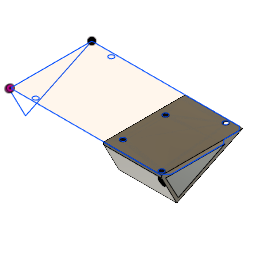
arduno wedge v1 (Autodesk Fusion 360 design; units mm, degrees)
Autodesk Fusion 360 part; units mm, degrees
(part 1 of 2)
sketch "dimensioniMega" plane through (-257.4607, -81.6493, 0) normal (0, 0, 1) x (1, 0, 0)
  line L0 (356.4838, 123.144) -> (359.0229, 120.6049)
  line L1 (359.0229, 120.6049) -> (359.0229, 86.3482)
  line L2 (258.4956, 82.5395) -> (258.2417, 82.5818)
  line L3 (258.2417, 82.5818) -> (258.0089, 82.6665)
  line L4 (258.4956, 135.8395) -> (353.9447, 135.8395)
  line L5 (257.7973, 135.5433) -> (258.0089, 135.6914)
  line L6 (356.4838, 133.3004) -> (356.4838, 123.144)
  line L7 (355.9971, 82.6665) -> (355.7432, 82.5818)
  line L8 (257.7973, 82.8357) -> (257.6281, 83.0473)
  line L9 (257.5434, 83.2801) -> (257.5011, 83.534)
  line L10 (359.0229, 86.3482) -> (356.4838, 83.8091)
  line L11 (355.4893, 82.5395) -> (258.4956, 82.5395)
  line L12 (257.5434, 135.0989) -> (257.6281, 135.3317)
  line L13 (258.0089, 135.6914) -> (258.2417, 135.7972)
  line L14 (257.5011, 134.8239) -> (257.5434, 135.0989)
  line L15 (257.6281, 135.3317) -> (257.7973, 135.5433)
  line L16 (356.4626, 83.2801) -> (356.3568, 83.0473)
  line L17 (356.4838, 83.8091) -> (356.4838, 83.534)
  line L18 (355.7432, 82.5818) -> (355.4893, 82.5395)
  line L19 (356.4838, 83.534) -> (356.4626, 83.2801)
  line L20 (258.0089, 82.6665) -> (257.7973, 82.8357)
  line L21 (258.2417, 135.7972) -> (258.4956, 135.8395)
  line L22 (257.5011, 83.534) -> (257.5011, 134.8239)
  line L23 (356.3568, 83.0473) -> (356.2087, 82.8357)
  line L24 (353.9447, 135.8395) -> (356.4838, 133.3004)
  line L25 (257.6281, 83.0473) -> (257.5434, 83.2801)
  line L26 (356.2087, 82.8357) -> (355.9971, 82.6665)
  line L27 (269.889, 85.3923) -> (269.879, 85.3375)
  line L28 (272.1711, 83.6333) -> (272.2211, 83.6587)
  line L29 (271.9631, 83.5492) -> (272.0162, 83.5675)
  line L30 (271.5223, 83.4715) -> (271.5783, 83.4744)
  line L31 (274.3429, 133.3561) -> (274.34, 133.4118)
  line L32 (271.3548, 83.4744) -> (271.4105, 83.4715)
  line L33 (274.3197, 133.5776) -> (274.3092, 133.6323)
  line L34 (273.0586, 84.8548) -> (273.0655, 84.9105)
  line L35 (274.3092, 133.6323) -> (274.2967, 133.6866)
  line L36 (274.2284, 133.8986) -> (274.2068, 133.95)
  line L37 (274.3284, 133.5226) -> (274.3197, 133.5776)
  line L38 (271.1342, 83.5051) -> (271.189, 83.4946)
  line L39 (272.7993, 84.1794) -> (272.8299, 84.2265)
  line L40 (272.1202, 83.6095) -> (272.1711, 83.6333)
  line L41 (270.1718, 84.1244) -> (270.2056, 84.0801)
  line L42 (269.9667, 85.6595) -> (269.9474, 85.6072)
  line L43 (273.0655, 84.9105) -> (273.0703, 84.9664)
  line L44 (271.189, 83.4946) -> (271.244, 83.4859)
  line L45 (272.2702, 83.686) -> (272.3183, 83.7149)
  line L46 (272.9115, 84.3737) -> (272.9352, 84.4245)
  line L47 (272.9956, 84.5817) -> (273.012, 84.6354)
  line L48 (274.34, 133.4118) -> (274.3351, 133.4673)
  line L49 (273.012, 84.6354) -> (273.0265, 84.6896)
  line L50 (272.8299, 84.2265) -> (272.8588, 84.2746)
  line L51 (273.0703, 84.9664) -> (273.0733, 85.0225)
  line L52 (273.0498, 84.7994) -> (273.0586, 84.8548)
  line L53 (272.5832, 83.9218) -> (272.6229, 83.9615)
  line L54 (272.6612, 84.0026) -> (272.698, 84.045)
  line L55 (273.0733, 85.0225) -> (273.0743, 85.0786)
  line L56 (271.7454, 83.4949) -> (271.8005, 83.5057)
  line L57 (271.244, 83.4859) -> (271.2993, 83.4792)
  line L58 (274.2824, 133.7405) -> (274.2663, 133.7938)
  line L59 (271.4105, 83.4715) -> (271.4662, 83.4705)
  line L60 (274.2663, 133.7938) -> (274.2482, 133.8465)
  line L61 (272.9773, 84.5286) -> (272.9956, 84.5817)
  line L62 (271.69, 83.4862) -> (271.7454, 83.4949)
  line L63 (272.5422, 83.8836) -> (272.5832, 83.9218)
  line L64 (271.6343, 83.4793) -> (271.69, 83.4862)
  line L65 (272.886, 84.3237) -> (272.9115, 84.3737)
  line L66 (271.0799, 83.5176) -> (271.1342, 83.5051)
  line L67 (272.4998, 83.8467) -> (272.5422, 83.8836)
  line L68 (273.0265, 84.6896) -> (273.0391, 84.7443)
  line L69 (272.2211, 83.6587) -> (272.2702, 83.686)
  line L70 (272.9572, 84.4762) -> (272.9773, 84.5286)
  line L71 (272.7671, 84.1334) -> (272.7993, 84.1794)
  line L72 (271.5783, 83.4744) -> (271.6343, 83.4793)
  line L73 (270.6196, 83.7114) -> (270.6675, 83.6829)
  line L74 (274.2967, 133.6866) -> (274.2824, 133.7405)
  line L75 (272.4562, 83.8114) -> (272.4998, 83.8467)
  line L76 (269.8688, 84.8933) -> (269.8762, 84.8381)
  line L77 (270.9728, 83.5481) -> (271.0261, 83.5319)
  line L78 (272.8588, 84.2746) -> (272.886, 84.3237)
  line L79 (272.7334, 84.0886) -> (272.7671, 84.1334)
  line L80 (274.3438, 133.3004) -> (274.3429, 133.3561)
  line L81 (274.3351, 133.4673) -> (274.3284, 133.5226)
  line L82 (271.2993, 83.4792) -> (271.3548, 83.4744)
  line L83 (272.698, 84.045) -> (272.7334, 84.0886)
  line L84 (272.4114, 83.7776) -> (272.4562, 83.8114)
  line L85 (273.0391, 84.7443) -> (273.0498, 84.7994)
  line L86 (272.3654, 83.7454) -> (272.4114, 83.7776)
  line L87 (271.8552, 83.5183) -> (271.9094, 83.5328)
  line L88 (271.9094, 83.5328) -> (271.9631, 83.5492)
  line L89 (271.0261, 83.5319) -> (271.0799, 83.5176)
  line L90 (273.6899, 134.5948) -> (273.6445, 134.6271)
  line L91 (273.6445, 134.6271) -> (273.598, 134.6578)
  line L92 (271.7227, 134.5494) -> (271.6801, 134.5135)
  line L93 (273.8191, 134.4888) -> (273.7773, 134.5256)
  line L94 (272.3183, 83.7149) -> (272.3654, 83.7454)
  line L95 (271.4662, 83.4705) -> (271.5223, 83.4715)
  line L96 (271.3884, 134.1783) -> (271.3588, 134.1311)
  line L97 (272.6229, 83.9615) -> (272.6612, 84.0026)
  line L98 (271.5599, 134.3974) -> (271.5226, 134.356)
  line L99 (274.1315, 134.0991) -> (274.103, 134.147)
  line L100 (272.4768, 134.8875) -> (272.422, 134.8776)
  line L101 (273.14, 134.8569) -> (273.0858, 134.8699)
  line L102 (272.532, 134.8955) -> (272.4768, 134.8875)
  line L103 (273.5505, 134.6868) -> (273.5019, 134.7142)
  line L104 (272.81, 134.9068) -> (272.7543, 134.9084)
  line L105 (274.2482, 133.8465) -> (274.2284, 133.8986)
  line L106 (272.0686, 83.5876) -> (272.1202, 83.6095)
  line L107 (271.3588, 134.1311) -> (271.3308, 134.0829)
  line L108 (273.8988, 134.4109) -> (273.8596, 134.4506)
  line L109 (272.9352, 84.4245) -> (272.9572, 84.4762)
  line L110 (271.3308, 134.0829) -> (271.3046, 134.0338)
  line L111 (271.3046, 134.0338) -> (271.28, 133.9838)
  line L112 (273.9729, 134.3277) -> (273.9366, 134.37)
  line L113 (271.6387, 134.4762) -> (271.5986, 134.4375)
  line L114 (273.8596, 134.4506) -> (273.8191, 134.4888)
  line L115 (272.5873, 134.9016) -> (272.532, 134.8955)
  line L116 (272.26, 134.8365) -> (272.2071, 134.8191)
  line L117 (272.0162, 83.5675) -> (272.0686, 83.5876)
  line L118 (273.5019, 134.7142) -> (273.4525, 134.7399)
  line L119 (271.905, 134.6773) -> (271.8578, 134.6477)
  line L120 (273.4525, 134.7399) -> (273.4022, 134.7639)
  line L121 (274.0411, 134.2396) -> (274.0077, 134.2843)
  line L122 (273.7342, 134.561) -> (273.6899, 134.5948)
  line L123 (272.0023, 134.7315) -> (271.9532, 134.7053)
  line L124 (273.2468, 134.8251) -> (273.1936, 134.8419)
  line L125 (272.3675, 134.8658) -> (272.3135, 134.8521)
  line L126 (271.5226, 134.356) -> (271.4868, 134.3134)
  line L127 (273.9366, 134.37) -> (273.8988, 134.4109)
  line L128 (272.6429, 134.9058) -> (272.5873, 134.9016)
  line L129 (271.7666, 134.5837) -> (271.7227, 134.5494)
  line L130 (272.1032, 134.7789) -> (272.0524, 134.7561)
  line L131 (271.8117, 134.6165) -> (271.7666, 134.5837)
  line L132 (273.7773, 134.5256) -> (273.7342, 134.561)
  line L133 (272.9763, 134.8904) -> (272.921, 134.8978)
  line L134 (272.8656, 134.9033) -> (272.81, 134.9068)
  line L135 (272.6986, 134.9081) -> (272.6429, 134.9058)
  line L136 (274.0077, 134.2843) -> (273.9729, 134.3277)
  line L137 (271.8005, 83.5057) -> (271.8552, 83.5183)
  line L138 (273.2993, 134.8065) -> (273.2468, 134.8251)
  line L139 (274.2068, 133.95) -> (274.1834, 134.0005)
  line L140 (272.0524, 134.7561) -> (272.0023, 134.7315)
  line L141 (273.4022, 134.7639) -> (273.3511, 134.7861)
  line L142 (272.3135, 134.8521) -> (272.26, 134.8365)
  line L143 (274.0728, 134.1938) -> (274.0411, 134.2396)
  line L144 (274.1834, 134.0005) -> (274.1583, 134.0503)
  line L145 (272.921, 134.8978) -> (272.8656, 134.9033)
  line L146 (274.1583, 134.0503) -> (274.1315, 134.0991)
  line L147 (272.2071, 134.8191) -> (272.1548, 134.7999)
  line L148 (271.9532, 134.7053) -> (271.905, 134.6773)
  line L149 (272.7543, 134.9084) -> (272.6986, 134.9081)
  line L150 (272.1548, 134.7999) -> (272.1032, 134.7789)
  line L151 (274.103, 134.147) -> (274.0728, 134.1938)
  line L152 (273.1936, 134.8419) -> (273.14, 134.8569)
  line L153 (271.8578, 134.6477) -> (271.8117, 134.6165)
  line L154 (271.5986, 134.4375) -> (271.5599, 134.3974)
  line L155 (273.0858, 134.8699) -> (273.0312, 134.8811)
  line L156 (271.4868, 134.3134) -> (271.4524, 134.2695)
  line L157 (272.422, 134.8776) -> (272.3675, 134.8658)
  line L158 (271.4524, 134.2695) -> (271.4196, 134.2245)
  line L159 (271.4196, 134.2245) -> (271.3884, 134.1783)
  line L160 (273.0312, 134.8811) -> (272.9763, 134.8904)
  line L161 (273.3511, 134.7861) -> (273.2993, 134.8065)
  line L162 (273.598, 134.6578) -> (273.5505, 134.6868)
  line L163 (271.6801, 134.5135) -> (271.6387, 134.4762)
  line L164 (271.5105, 132.2589) -> (271.5473, 132.217)
  line L165 (271.7084, 132.0632) -> (271.7519, 132.0284)
  line L166 (273.1248, 131.7401) -> (273.179, 131.7546)
  line L167 (271.1345, 133.4488) -> (271.1303, 133.3932)
  line L168 (272.9038, 131.7011) -> (272.9595, 131.708)
  line L169 (272.5136, 131.7077) -> (272.5689, 131.701)
  line L170 (272.5689, 131.701) -> (272.6244, 131.6962)
  line L171 (271.211, 132.7894) -> (271.2296, 132.7369)
  line L172 (271.7519, 132.0284) -> (271.7965, 131.9951)
  line L173 (271.8892, 131.9332) -> (271.937, 131.9047)
  line L174 (271.184, 133.7226) -> (271.1703, 133.6686)
  line L175 (271.5856, 132.1765) -> (271.6252, 132.1374)
  line L176 (271.1662, 132.9503) -> (271.1793, 132.8962)
  line L177 (271.1293, 133.2261) -> (271.1329, 133.1705)
  line L178 (271.3784, 132.4381) -> (271.409, 132.3916)
  line L179 (271.8423, 131.9633) -> (271.8892, 131.9332)
  line L180 (272.2956, 131.7537) -> (272.3495, 131.7394)
  line L181 (272.8479, 131.6962) -> (272.9038, 131.7011)
  line L182 (271.1793, 132.8962) -> (271.1942, 132.8425)
  line L183 (271.6252, 132.1374) -> (271.6661, 132.0996)
  line L184 (271.1303, 133.3932) -> (271.128, 133.3376)
  line L185 (271.1383, 133.1151) -> (271.1457, 133.0599)
  line L186 (271.1486, 133.5593) -> (271.1406, 133.5042)
  line L187 (271.128, 133.3376) -> (271.1277, 133.2818)
  line L188 (272.4038, 131.7269) -> (272.4585, 131.7164)
  line L189 (272.0862, 131.8293) -> (272.1375, 131.8077)
  line L190 (271.28, 133.9838) -> (271.2572, 133.9329)
  line L191 (271.1277, 133.2818) -> (271.1293, 133.2261)
  line L192 (271.2722, 132.6339) -> (271.2962, 132.5836)
  line L193 (271.5473, 132.217) -> (271.5856, 132.1765)
  line L194 (271.9859, 131.8778) -> (272.0356, 131.8527)
  line L195 (271.6661, 132.0996) -> (271.7084, 132.0632)
  line L196 (272.0356, 131.8527) -> (272.0862, 131.8293)
  line L197 (271.4413, 132.3462) -> (271.4752, 132.3019)
  line L198 (271.217, 133.829) -> (271.1996, 133.7761)
  line L199 (271.3493, 132.4857) -> (271.3784, 132.4381)
  line L200 (271.4752, 132.3019) -> (271.5105, 132.2589)
  line L201 (271.2296, 132.7369) -> (271.25, 132.685)
  line L202 (272.3495, 131.7394) -> (272.4038, 131.7269)
  line L203 (272.9595, 131.708) -> (273.015, 131.7167)
  line L204 (271.1942, 132.8425) -> (271.211, 132.7894)
  line L205 (271.1329, 133.1705) -> (271.1383, 133.1151)
  line L206 (271.409, 132.3916) -> (271.4413, 132.3462)
  line L207 (271.3219, 132.5342) -> (271.3493, 132.4857)
  line L208 (271.1406, 133.5042) -> (271.1345, 133.4488)
  line L209 (271.1703, 133.6686) -> (271.1585, 133.6141)
  line L210 (272.1375, 131.8077) -> (272.1896, 131.7879)
  line L211 (272.4585, 131.7164) -> (272.5136, 131.7077)
  line L212 (271.937, 131.9047) -> (271.9859, 131.8778)
  line L213 (271.155, 133.0049) -> (271.1662, 132.9503)
  line L214 (271.1457, 133.0599) -> (271.155, 133.0049)
  line L215 (272.68, 131.6933) -> (272.7357, 131.6923)
  line L216 (271.25, 132.685) -> (271.2722, 132.6339)
  line L217 (271.1585, 133.6141) -> (271.1486, 133.5593)
  line L218 (272.6244, 131.6962) -> (272.68, 131.6933)
  line L219 (271.2572, 133.9329) -> (271.2362, 133.8813)
  line L220 (271.1996, 133.7761) -> (271.184, 133.7226)
  line L221 (271.2362, 133.8813) -> (271.217, 133.829)
  line L222 (271.7965, 131.9951) -> (271.8423, 131.9633)
  line L223 (272.7918, 131.6933) -> (272.8479, 131.6962)
  line L224 (272.2423, 131.7699) -> (272.2956, 131.7537)
  line L225 (272.7357, 131.6923) -> (272.7918, 131.6933)
  line L226 (272.1896, 131.7879) -> (272.2423, 131.7699)
  line L227 (271.2962, 132.5836) -> (271.3219, 132.5342)
  line L228 (273.635, 131.9672) -> (273.6809, 131.9994)
  line L229 (273.3898, 131.8313) -> (273.4407, 131.8551)
  line L230 (273.7694, 132.0685) -> (273.8117, 132.1054)
  line L231 (273.2326, 131.771) -> (273.2857, 131.7893)
  line L232 (273.015, 131.7167) -> (273.0701, 131.7275)
  line L233 (273.5398, 131.9078) -> (273.5879, 131.9367)
  line L234 (273.5879, 131.9367) -> (273.635, 131.9672)
  line L235 (273.3381, 131.8094) -> (273.3898, 131.8313)
  line L236 (273.179, 131.7546) -> (273.2326, 131.771)
  line L237 (273.7258, 132.0332) -> (273.7694, 132.0685)
  line L238 (273.0701, 131.7275) -> (273.1248, 131.7401)
  line L239 (273.2857, 131.7893) -> (273.3381, 131.8094)
  line L240 (273.4407, 131.8551) -> (273.4907, 131.8805)
  line L241 (273.6809, 131.9994) -> (273.7258, 132.0332)
  line L242 (273.4907, 131.8805) -> (273.5398, 131.9078)
  line L243 (270.0105, 85.762) -> (269.9877, 85.7111)
  line L244 (270.3556, 83.9156) -> (270.3966, 83.8778)
  line L245 (269.9877, 85.7111) -> (269.9667, 85.6595)
  line L246 (270.1829, 86.0477) -> (270.1501, 86.0027)
  line L247 (269.879, 85.3375) -> (269.871, 85.2824)
  line L248 (270.1395, 84.1698) -> (270.1718, 84.1244)
  line L249 (269.8582, 85.06) -> (269.8598, 85.0043)
  line L250 (270.2904, 86.1756) -> (270.2531, 86.1342)
  line L251 (269.9246, 84.6207) -> (269.9414, 84.5676)
  line L252 (270.3966, 83.8778) -> (270.4388, 83.8415)
  line L253 (270.5728, 83.7415) -> (270.6196, 83.7114)
  line L254 (269.9474, 85.6072) -> (269.93, 85.5543)
  line L255 (269.871, 85.2824) -> (269.8649, 85.227)
  line L256 (269.9601, 84.5151) -> (269.9805, 84.4632)
  line L257 (270.2056, 84.0801) -> (270.241, 84.0371)
  line L258 (270.527, 83.7733) -> (270.5728, 83.7415)
  line L259 (270.2172, 86.0916) -> (270.1829, 86.0477)
  line L260 (270.7163, 83.656) -> (270.7661, 83.6309)
  line L261 (269.8649, 85.227) -> (269.8608, 85.1714)
  line L262 (270.0027, 84.4121) -> (270.0267, 84.3618)
  line L263 (269.8762, 84.8381) -> (269.8855, 84.7831)
  line L264 (270.8166, 83.6075) -> (270.868, 83.5859)
  line L265 (270.4823, 83.8066) -> (270.527, 83.7733)
  line L266 (269.8633, 84.9487) -> (269.8688, 84.8933)
  line L267 (270.0524, 84.3124) -> (270.0797, 84.2639)
  line L268 (270.035, 85.812) -> (270.0105, 85.762)
  line L269 (270.7661, 83.6309) -> (270.8166, 83.6075)
  line L270 (270.6675, 83.6829) -> (270.7163, 83.656)
  line L271 (269.93, 85.5543) -> (269.9145, 85.5008)
  line L272 (269.9145, 85.5008) -> (269.9008, 85.4468)
  line L273 (270.0892, 85.9093) -> (270.0613, 85.8611)
  line L274 (270.1189, 85.9565) -> (270.0892, 85.9093)
  line L275 (269.8608, 85.1714) -> (269.8585, 85.1158)
  line L276 (270.1501, 86.0027) -> (270.1189, 85.9565)
  line L277 (270.2531, 86.1342) -> (270.2172, 86.0916)
  line L278 (270.0267, 84.3618) -> (270.0524, 84.3124)
  line L279 (269.8585, 85.1158) -> (269.8582, 85.06)
  line L280 (269.9414, 84.5676) -> (269.9601, 84.5151)
  line L281 (269.8598, 85.0043) -> (269.8633, 84.9487)
  line L282 (269.8855, 84.7831) -> (269.8966, 84.7285)
  line L283 (269.9805, 84.4632) -> (270.0027, 84.4121)
  line L284 (270.1088, 84.2163) -> (270.1395, 84.1698)
  line L285 (269.9097, 84.6744) -> (269.9246, 84.6207)
  line L286 (270.868, 83.5859) -> (270.92, 83.5661)
  line L287 (269.9008, 85.4468) -> (269.889, 85.3923)
  line L288 (270.0613, 85.8611) -> (270.035, 85.812)
  line L289 (270.2778, 83.9952) -> (270.316, 83.9547)
  line L290 (270.92, 83.5661) -> (270.9728, 83.5481)
  line L291 (270.0797, 84.2639) -> (270.1088, 84.2163)
  line L292 (270.316, 83.9547) -> (270.3556, 83.9156)
  line L293 (269.8966, 84.7285) -> (269.9097, 84.6744)
  line L294 (322.5275, 91.4401) -> (322.4836, 91.4058)
  line L295 (321.8889, 90.194) -> (321.8886, 90.1382)
  line L296 (321.9402, 89.7526) -> (321.9551, 89.6989)
  line L297 (322.2361, 89.1583) -> (322.2714, 89.1153)
  line L298 (321.9779, 90.6854) -> (321.9605, 90.6325)
  line L299 (322.0109, 89.5414) -> (322.0331, 89.4903)
  line L300 (322.6187, 91.5041) -> (322.5726, 91.4729)
  line L301 (321.9095, 90.4157) -> (321.9015, 90.3606)
  line L302 (321.9271, 89.8068) -> (321.9402, 89.7526)
  line L303 (321.8912, 90.2496) -> (321.8889, 90.194)
  line L304 (321.9312, 90.525) -> (321.9194, 90.4705)
  line L305 (321.9905, 89.5933) -> (322.0109, 89.5414)
  line L306 (322.2835, 91.2125) -> (322.2477, 91.1698)
  line L307 (322.1805, 91.0809) -> (322.1493, 91.0347)
  line L308 (322.1102, 89.3421) -> (322.1393, 89.2945)
  line L309 (323.1829, 91.734) -> (323.1284, 91.7222)
  line L310 (322.8133, 91.6125) -> (322.7632, 91.588)
  line L311 (322.2714, 89.1153) -> (322.3082, 89.0735)
  line L312 (322.2477, 91.1698) -> (322.2133, 91.1259)
  line L313 (322.4836, 91.4058) -> (322.441, 91.3699)
  line L314 (322.1699, 89.248) -> (322.2022, 89.2026)
  line L315 (322.441, 91.3699) -> (322.3996, 91.3326)
  line L316 (321.9719, 89.6458) -> (321.9905, 89.5933)
  line L317 (321.9971, 90.7377) -> (321.9779, 90.6854)
  line L318 (321.8954, 90.3052) -> (321.8912, 90.2496)
  line L319 (321.9449, 90.579) -> (321.9312, 90.525)
  line L320 (323.2929, 91.752) -> (323.2377, 91.7439)
  line L321 (321.8886, 90.1382) -> (321.8902, 90.0826)
  line L322 (322.0331, 89.4903) -> (322.0571, 89.44)
  line L323 (322.0917, 90.9393) -> (322.0655, 90.8902)
  line L324 (324.8604, 89.3047) -> (324.8893, 89.3528)
  line L325 (322.7632, 91.588) -> (322.7141, 91.5617)
  line L326 (323.0209, 91.693) -> (322.968, 91.6756)
  line L327 (321.8938, 90.0269) -> (321.8992, 89.9715)
  line L328 (324.099, 88.6658) -> (324.1507, 88.6878)
  line L329 (322.3595, 91.2939) -> (322.3208, 91.2538)
  line L330 (322.1393, 89.2945) -> (322.1699, 89.248)
  line L331 (322.2022, 89.2026) -> (322.2361, 89.1583)
  line L332 (321.9194, 90.4705) -> (321.9095, 90.4157)
  line L333 (321.9551, 89.6989) -> (321.9719, 89.6458)
  line L334 (322.6659, 91.5337) -> (322.6187, 91.5041)
  line L335 (323.2377, 91.7439) -> (323.1829, 91.734)
  line L336 (322.5726, 91.4729) -> (322.5275, 91.4401)
  line L337 (322.2133, 91.1259) -> (322.1805, 91.0809)
  line L338 (322.9157, 91.6563) -> (322.8641, 91.6353)
  line L339 (322.3082, 89.0735) -> (322.3465, 89.0329)
  line L340 (322.3996, 91.3326) -> (322.3595, 91.2939)
  line L341 (323.1284, 91.7222) -> (323.0744, 91.7085)
  line L342 (322.1197, 90.9875) -> (322.0917, 90.9393)
  line L343 (323.0744, 91.7085) -> (323.0209, 91.693)
  line L344 (322.0655, 90.8902) -> (322.0409, 90.8402)
  line L345 (322.7141, 91.5617) -> (322.6659, 91.5337)
  line L346 (321.9015, 90.3606) -> (321.8954, 90.3052)
  line L347 (321.8902, 90.0826) -> (321.8938, 90.0269)
  line L348 (321.8992, 89.9715) -> (321.9066, 89.9163)
  line L349 (321.9159, 89.8613) -> (321.9271, 89.8068)
  line L350 (322.0181, 90.7893) -> (321.9971, 90.7377)
  line L351 (322.968, 91.6756) -> (322.9157, 91.6563)
  line L352 (321.9605, 90.6325) -> (321.9449, 90.579)
  line L353 (323.7204, 88.5644) -> (323.7759, 88.5732)
  line L354 (323.9399, 88.611) -> (323.9935, 88.6274)
  line L355 (325.0424, 89.7136) -> (325.0569, 89.7678)
  line L356 (322.7468, 88.7343) -> (322.7965, 88.7091)
  line L357 (323.0032, 88.6263) -> (323.0565, 88.6101)
  line L358 (324.3007, 88.7642) -> (324.3488, 88.7931)
  line L359 (325.026, 89.6599) -> (325.0424, 89.7136)
  line L360 (322.4693, 88.9197) -> (322.5128, 88.8848)
  line L361 (323.1104, 88.5958) -> (323.1647, 88.5834)
  line L362 (323.4409, 88.5497) -> (323.4966, 88.5487)
  line L363 (322.5128, 88.8848) -> (322.5574, 88.8515)
  line L364 (324.4867, 88.8896) -> (324.5303, 88.9249)
  line L365 (324.9165, 89.4019) -> (324.942, 89.4519)
  line L366 (323.831, 88.5839) -> (323.8857, 88.5965)
  line L367 (323.4966, 88.5487) -> (323.5527, 88.5497)
  line L368 (322.8471, 88.6857) -> (322.8984, 88.6641)
  line L369 (324.5726, 88.9618) -> (324.6137, 89.0001)
  line L370 (323.0565, 88.6101) -> (323.1104, 88.5958)
  line L371 (322.3465, 89.0329) -> (322.3861, 88.9938)
  line L372 (324.3488, 88.7931) -> (324.3959, 88.8236)
  line L373 (323.2194, 88.5728) -> (323.2744, 88.5641)
  line L374 (324.6917, 89.0808) -> (324.7285, 89.1232)
  line L375 (322.8984, 88.6641) -> (322.9505, 88.6443)
  line L376 (322.9505, 88.6443) -> (323.0032, 88.6263)
  line L377 (324.6534, 89.0397) -> (324.6917, 89.0808)
  line L378 (324.1507, 88.6878) -> (324.2016, 88.7115)
  line L379 (324.7976, 89.2116) -> (324.8298, 89.2576)
  line L380 (324.8893, 89.3528) -> (324.9165, 89.4019)
  line L381 (324.4418, 88.8558) -> (324.4867, 88.8896)
  line L382 (324.2016, 88.7115) -> (324.2516, 88.737)
  line L383 (322.6979, 88.7611) -> (322.7468, 88.7343)
  line L384 (323.2744, 88.5641) -> (323.3298, 88.5574)
  line L385 (324.2516, 88.737) -> (324.3007, 88.7642)
  line L386 (322.6501, 88.7896) -> (322.6979, 88.7611)
  line L387 (323.1647, 88.5834) -> (323.2194, 88.5728)
  line L388 (323.8857, 88.5965) -> (323.9399, 88.611)
  line L389 (322.427, 88.956) -> (322.4693, 88.9197)
  line L390 (323.6088, 88.5526) -> (323.6647, 88.5575)
  line L391 (324.3959, 88.8236) -> (324.4418, 88.8558)
  line L392 (324.8298, 89.2576) -> (324.8604, 89.3047)
  line L393 (323.9935, 88.6274) -> (324.0466, 88.6457)
  line L394 (323.3298, 88.5574) -> (323.3853, 88.5526)
  line L395 (322.5574, 88.8515) -> (322.6032, 88.8197)
  line L396 (323.7759, 88.5732) -> (323.831, 88.5839)
  line L397 (324.942, 89.4519) -> (324.9657, 89.5027)
  line L398 (325.0696, 89.8225) -> (325.0803, 89.8776)
  line L399 (324.6137, 89.0001) -> (324.6534, 89.0397)
  line L400 (322.7965, 88.7091) -> (322.8471, 88.6857)
  line L401 (324.0466, 88.6457) -> (324.099, 88.6658)
  line L402 (322.6032, 88.8197) -> (322.6501, 88.7896)
  line L403 (324.7285, 89.1232) -> (324.7638, 89.1668)
  line L404 (325.0569, 89.7678) -> (325.0696, 89.8225)
  line L405 (323.5527, 88.5497) -> (323.6088, 88.5526)
  line L406 (324.9876, 89.5544) -> (325.0077, 89.6068)
  line L407 (325.0077, 89.6068) -> (325.026, 89.6599)
  line L408 (323.3853, 88.5526) -> (323.4409, 88.5497)
  line L409 (324.5303, 88.9249) -> (324.5726, 88.9618)
  line L410 (324.9657, 89.5027) -> (324.9876, 89.5544)
  line L411 (324.7638, 89.1668) -> (324.7976, 89.2116)
  line L412 (324.9893, 118.664) -> (324.9677, 118.7153)
  line L413 (324.0602, 119.5719) -> (324.0077, 119.5905)
  line L414 (324.0077, 119.5905) -> (323.9545, 119.6073)
  line L415 (324.112, 119.5515) -> (324.0602, 119.5719)
  line L416 (321.9779, 118.5944) -> (321.9605, 118.5415)
  line L417 (322.0109, 117.4504) -> (322.0331, 117.3993)
  line L418 (322.0331, 117.3993) -> (322.0571, 117.349)
  line L419 (323.7921, 119.6465) -> (323.7372, 119.6558)
  line L420 (322.5275, 119.3491) -> (322.4836, 119.3147)
  line L421 (323.8467, 119.6353) -> (323.7921, 119.6465)
  line L422 (324.3114, 119.4522) -> (324.2628, 119.4796)
  line L423 (322.0571, 117.349) -> (322.0828, 117.2996)
  line L424 (323.6647, 88.5575) -> (323.7204, 88.5644)
  line L425 (325.0893, 118.288) -> (325.0806, 118.343)
  line L426 (322.3861, 88.9938) -> (322.427, 88.956)
  line L427 (324.8638, 118.9123) -> (324.8337, 118.9592)
  line L428 (324.2134, 119.5053) -> (324.1631, 119.5293)
  line L429 (324.5382, 119.291) -> (324.4951, 119.3264)
  line L430 (324.6597, 119.1763) -> (324.6205, 119.2159)
  line L431 (324.4508, 119.3602) -> (324.4054, 119.3925)
  line L432 (325.0091, 118.6119) -> (324.9893, 118.664)
  line L433 (324.4951, 119.3264) -> (324.4508, 119.3602)
  line L434 (323.9009, 119.6223) -> (323.8467, 119.6353)
  line L435 (324.8337, 118.9592) -> (324.8019, 119.005)
  line L436 (325.0433, 118.5059) -> (325.0272, 118.5592)
  line L437 (323.3482, 119.667) -> (323.2929, 119.6609)
  line L438 (324.8924, 118.8645) -> (324.8638, 118.9123)
  line L439 (325.0806, 118.343) -> (325.0701, 118.3977)
  line L440 (324.6974, 119.1354) -> (324.6597, 119.1763)
  line L441 (325.1047, 118.0658) -> (325.1037, 118.1215)
  line L442 (324.6205, 119.2159) -> (324.58, 119.2542)
  line L443 (324.3589, 119.4232) -> (324.3114, 119.4522)
  line L444 (324.8019, 119.005) -> (324.7686, 119.0496)
  line L445 (323.9545, 119.6073) -> (323.9009, 119.6223)
  line L446 (325.0803, 89.8776) -> (325.0891, 89.933)
  line L447 (325.1009, 118.1771) -> (325.096, 118.2327)
  line L448 (324.7686, 119.0496) -> (324.7338, 119.0931)
  line L449 (325.0272, 118.5592) -> (325.0091, 118.6119)
  line L450 (325.0576, 118.452) -> (325.0433, 118.5059)
  line L451 (322.1493, 118.9437) -> (322.1197, 118.8965)
  line L452 (322.0181, 118.6983) -> (321.9971, 118.6467)
  line L453 (325.1037, 118.1215) -> (325.1009, 118.1771)
  line L454 (324.9443, 118.7659) -> (324.9192, 118.8156)
  line L455 (325.1008, 90.0446) -> (325.1037, 90.1007)
  line L456 (323.7372, 119.6558) -> (323.6819, 119.6632)
  line L457 (324.9677, 118.7153) -> (324.9443, 118.7659)
  line L458 (325.0701, 118.3977) -> (325.0576, 118.452)
  line L459 (325.096, 118.2327) -> (325.0893, 118.288)
  line L460 (324.4054, 119.3925) -> (324.3589, 119.4232)
  line L461 (325.1037, 90.1007) -> (325.1047, 90.1568)
  line L462 (324.9192, 118.8156) -> (324.8924, 118.8645)
  line L463 (325.0891, 89.933) -> (325.0959, 89.9887)
  line L464 (324.1631, 119.5293) -> (324.112, 119.5515)
  line L465 (324.58, 119.2542) -> (324.5382, 119.291)
  line L466 (321.9905, 117.5022) -> (322.0109, 117.4504)
  line L467 (325.0959, 89.9887) -> (325.1008, 90.0446)
  line L468 (324.7338, 119.0931) -> (324.6974, 119.1354)
  line L469 (324.2628, 119.4796) -> (324.2134, 119.5053)
  line L470 (321.8886, 118.0472) -> (321.8902, 117.9915)
  line L471 (321.8902, 117.9915) -> (321.8938, 117.9359)
  line L472 (321.9449, 118.488) -> (321.9312, 118.434)
  line L473 (322.6187, 119.4131) -> (322.5726, 119.3819)
  line L474 (321.8938, 117.9359) -> (321.8992, 117.8805)
  line L475 (321.9159, 117.7703) -> (321.9271, 117.7157)
  line L476 (321.8889, 118.1029) -> (321.8886, 118.0472)
  line L477 (322.3208, 119.1628) -> (322.2835, 119.1214)
  line L478 (323.6265, 119.6686) -> (323.5709, 119.6722)
  line L479 (321.9271, 117.7157) -> (321.9402, 117.6616)
  line L480 (321.9312, 118.434) -> (321.9194, 118.3795)
  line L481 (323.0744, 119.6175) -> (323.0209, 119.6019)
  line L482 (322.7141, 119.4707) -> (322.6659, 119.4427)
  line L483 (323.0209, 119.6019) -> (322.968, 119.5845)
  line L484 (321.9015, 118.2696) -> (321.8954, 118.2142)
  line L485 (322.0917, 118.8483) -> (322.0655, 118.7992)
  line L486 (323.1284, 119.6312) -> (323.0744, 119.6175)
  line L487 (322.3996, 119.2416) -> (322.3595, 119.2029)
  line L488 (321.9605, 118.5415) -> (321.9449, 118.488)
  line L489 (321.8912, 118.1586) -> (321.8889, 118.1029)
  line L490 (322.6659, 119.4427) -> (322.6187, 119.4131)
  line L491 (323.6819, 119.6632) -> (323.6265, 119.6686)
  line L492 (322.3595, 119.2029) -> (322.3208, 119.1628)
  line L493 (322.2477, 119.0788) -> (322.2133, 119.0349)
  line L494 (321.8992, 117.8805) -> (321.9066, 117.8252)
  line L495 (323.1829, 119.643) -> (323.1284, 119.6312)
  line L496 (322.8641, 119.5443) -> (322.8133, 119.5215)
  line L497 (322.1197, 118.8965) -> (322.0917, 118.8483)
  line L498 (322.8133, 119.5215) -> (322.7632, 119.4969)
  line L499 (322.2133, 119.0349) -> (322.1805, 118.9899)
  line L500 (322.5726, 119.3819) -> (322.5275, 119.3491)
  line L501 (321.9066, 117.8252) -> (321.9159, 117.7703)
  line L502 (321.9402, 117.6616) -> (321.9551, 117.6079)
  line L503 (321.9551, 117.6079) -> (321.9719, 117.5548)
  line L504 (321.9194, 118.3795) -> (321.9095, 118.3247)
  line L505 (322.9157, 119.5653) -> (322.8641, 119.5443)
  line L506 (321.9719, 117.5548) -> (321.9905, 117.5022)
  line L507 (323.4595, 119.6735) -> (323.4038, 119.6712)
  line L508 (324.9165, 117.3108) -> (324.942, 117.3608)
  line L509 (323.5152, 119.6738) -> (323.4595, 119.6735)
  line L510 (323.2377, 119.6529) -> (323.1829, 119.643)
  line L511 (321.8954, 118.2142) -> (321.8912, 118.1586)
  line L512 (322.1805, 118.9899) -> (322.1493, 118.9437)
  line L513 (321.9971, 118.6467) -> (321.9779, 118.5944)
  line L514 (322.4836, 119.3147) -> (322.441, 119.2789)
  line L515 (322.7632, 119.4969) -> (322.7141, 119.4707)
  line L516 (322.441, 119.2789) -> (322.3996, 119.2416)
  line L517 (322.0409, 118.7491) -> (322.0181, 118.6983)
  line L518 (323.5709, 119.6722) -> (323.5152, 119.6738)
  line L519 (322.0828, 117.2996) -> (322.1102, 117.251)
  line L520 (322.0655, 118.7992) -> (322.0409, 118.7491)
  line L521 (321.9095, 118.3247) -> (321.9015, 118.2696)
  line L522 (322.968, 119.5845) -> (322.9157, 119.5653)
  line L523 (322.2835, 119.1214) -> (322.2477, 119.0788)
  line L524 (323.4038, 119.6712) -> (323.3482, 119.667)
  line L525 (323.2929, 119.6609) -> (323.2377, 119.6529)
  line L526 (323.8857, 116.5055) -> (323.9399, 116.52)
  line L527 (323.7759, 116.4821) -> (323.831, 116.4928)
  line L528 (322.8471, 116.5947) -> (322.8984, 116.5731)
  line L529 (323.5527, 116.4587) -> (323.6088, 116.4616)
  line L530 (323.6647, 116.4665) -> (323.7204, 116.4733)
  line L531 (324.942, 117.3608) -> (324.9657, 117.4117)
  line L532 (323.3853, 116.4616) -> (323.4409, 116.4587)
  line L533 (322.3465, 116.9419) -> (322.3861, 116.9027)
  line L534 (323.6088, 116.4616) -> (323.6647, 116.4665)
  line L535 (324.1507, 116.5967) -> (324.2016, 116.6204)
  line L536 (323.9399, 116.52) -> (323.9935, 116.5364)
  line L537 (322.2714, 117.0242) -> (322.3082, 116.9824)
  line L538 (322.6979, 116.6701) -> (322.7468, 116.6432)
  line L539 (322.2361, 117.0673) -> (322.2714, 117.0242)
  line L540 (323.1104, 116.5048) -> (323.1647, 116.4923)
  line L541 (323.1647, 116.4923) -> (323.2194, 116.4818)
  line L542 (323.0032, 116.5353) -> (323.0565, 116.5191)
  line L543 (322.1393, 117.2035) -> (322.1699, 117.157)
  line L544 (324.099, 116.5748) -> (324.1507, 116.5967)
  line L545 (324.7285, 117.0321) -> (324.7638, 117.0757)
  line L546 (322.1102, 117.251) -> (322.1393, 117.2035)
  line L547 (322.5128, 116.7938) -> (322.5574, 116.7605)
  line L548 (324.5303, 116.8339) -> (324.5726, 116.8707)
  line L549 (324.7638, 117.0757) -> (324.7976, 117.1206)
  line L550 (323.4966, 116.4577) -> (323.5527, 116.4587)
  line L551 (322.2022, 117.1116) -> (322.2361, 117.0673)
  line L552 (322.427, 116.865) -> (322.4693, 116.8286)
  line L553 (324.8604, 117.2136) -> (324.8893, 117.2617)
  line L554 (323.7204, 116.4733) -> (323.7759, 116.4821)
  line L555 (323.4409, 116.4587) -> (323.4966, 116.4577)
  line L556 (322.4693, 116.8286) -> (322.5128, 116.7938)
  line L557 (324.4867, 116.7986) -> (324.5303, 116.8339)
  line L558 (323.3298, 116.4664) -> (323.3853, 116.4616)
  line L559 (322.3082, 116.9824) -> (322.3465, 116.9419)
  line L560 (322.6501, 116.6986) -> (322.6979, 116.6701)
  line L561 (323.0565, 116.5191) -> (323.1104, 116.5048)
  line L562 (322.5574, 116.7605) -> (322.6032, 116.7287)
  line L563 (322.7965, 116.6181) -> (322.8471, 116.5947)
  line L564 (323.9935, 116.5364) -> (324.0466, 116.5547)
  line L565 (324.3007, 116.6731) -> (324.3488, 116.702)
  line L566 (324.4418, 116.7648) -> (324.4867, 116.7986)
  line L567 (324.2516, 116.6459) -> (324.3007, 116.6731)
  line L568 (324.5726, 116.8707) -> (324.6137, 116.909)
  line L569 (324.3488, 116.702) -> (324.3959, 116.7326)
  line L570 (323.2194, 116.4818) -> (323.2744, 116.4731)
  line L571 (322.7468, 116.6432) -> (322.7965, 116.6181)
  line L572 (324.7976, 117.1206) -> (324.8298, 117.1666)
  line L573 (324.6137, 116.909) -> (324.6534, 116.9487)
  line L574 (324.6917, 116.9898) -> (324.7285, 117.0321)
  line L575 (322.3861, 116.9027) -> (322.427, 116.865)
  line L576 (324.8893, 117.2617) -> (324.9165, 117.3108)
  line L577 (324.0466, 116.5547) -> (324.099, 116.5748)
  line L578 (323.831, 116.4928) -> (323.8857, 116.5055)
  line L579 (322.9505, 116.5533) -> (323.0032, 116.5353)
  line L580 (323.2744, 116.4731) -> (323.3298, 116.4664)
  line L581 (324.6534, 116.9487) -> (324.6917, 116.9898)
  line L582 (322.8984, 116.5731) -> (322.9505, 116.5533)
  line L583 (324.2016, 116.6204) -> (324.2516, 116.6459)
  line L584 (324.3959, 116.7326) -> (324.4418, 116.7648)
  line L585 (348.2335, 134.7861) -> (348.1816, 134.8065)
  line L586 (324.8298, 117.1666) -> (324.8604, 117.2136)
  line L587 (347.9682, 134.8699) -> (347.9136, 134.8811)
  line L588 (322.1699, 117.157) -> (322.2022, 117.1116)
  line L589 (322.6032, 116.7287) -> (322.6501, 116.6986)
  line L590 (347.0372, 134.7999) -> (346.9856, 134.7789)
  line L591 (346.082, 133.7761) -> (346.0664, 133.7226)
  line L592 (347.5253, 134.9058) -> (347.4697, 134.9016)
  line L593 (325.0077, 117.5158) -> (325.026, 117.5689)
  line L594 (348.8189, 134.37) -> (348.7812, 134.4109)
  line L595 (348.1291, 134.8251) -> (348.076, 134.8419)
  line L596 (349.2021, 133.5776) -> (349.1916, 133.6323)
  line L597 (348.8553, 134.3277) -> (348.8189, 134.37)
  line L598 (348.7015, 134.4888) -> (348.6596, 134.5256)
  line L599 (348.2846, 134.7639) -> (348.2335, 134.7861)
  line L600 (348.1816, 134.8065) -> (348.1291, 134.8251)
  line L601 (325.1037, 118.0097) -> (325.1047, 118.0658)
  line L602 (348.8901, 134.2843) -> (348.8553, 134.3277)
  line L603 (348.9234, 134.2396) -> (348.8901, 134.2843)
  line L604 (347.4697, 134.9016) -> (347.4143, 134.8955)
  line L605 (347.9136, 134.8811) -> (347.8586, 134.8904)
  line L606 (325.0959, 117.8977) -> (325.1008, 117.9536)
  line L607 (325.026, 117.5689) -> (325.0424, 117.6225)
  line L608 (348.7812, 134.4109) -> (348.742, 134.4506)
  line L609 (349.0892, 133.95) -> (349.0658, 134.0005)
  line L610 (325.0891, 117.842) -> (325.0959, 117.8977)
  line L611 (347.748, 134.9033) -> (347.6924, 134.9068)
  line L612 (349.2252, 133.3561) -> (349.2223, 133.4118)
  line L613 (348.9853, 134.147) -> (348.9552, 134.1938)
  line L614 (347.3592, 134.8875) -> (347.3044, 134.8776)
  line L615 (348.0223, 134.8569) -> (347.9682, 134.8699)
  line L616 (347.6924, 134.9068) -> (347.6367, 134.9084)
  line L617 (324.9876, 117.4634) -> (325.0077, 117.5158)
  line L618 (324.9657, 117.4117) -> (324.9876, 117.4634)
  line L619 (347.8034, 134.8978) -> (347.748, 134.9033)
  line L620 (349.2175, 133.4673) -> (349.2108, 133.5226)
  line L621 (325.0569, 117.6768) -> (325.0696, 117.7315)
  line L622 (347.5809, 134.9081) -> (347.5253, 134.9058)
  line L623 (349.0658, 134.0005) -> (349.0407, 134.0503)
  line L624 (347.4143, 134.8955) -> (347.3592, 134.8875)
  line L625 (325.1008, 117.9536) -> (325.1037, 118.0097)
  line L626 (349.2108, 133.5226) -> (349.2021, 133.5776)
  line L627 (349.1648, 133.7405) -> (349.1486, 133.7938)
  line L628 (347.8586, 134.8904) -> (347.8034, 134.8978)
  line L629 (325.0696, 117.7315) -> (325.0803, 117.7866)
  line L630 (349.2262, 133.3004) -> (349.2252, 133.3561)
  line L631 (348.3349, 134.7399) -> (348.2846, 134.7639)
  line L632 (348.5723, 134.5948) -> (348.5269, 134.6271)
  line L633 (349.1108, 133.8986) -> (349.0892, 133.95)
  line L634 (349.0407, 134.0503) -> (349.0138, 134.0991)
  line L635 (348.9552, 134.1938) -> (348.9234, 134.2396)
  line L636 (349.1306, 133.8465) -> (349.1108, 133.8986)
  line L637 (348.4328, 134.6868) -> (348.3843, 134.7142)
  line L638 (347.6367, 134.9084) -> (347.5809, 134.9081)
  line L639 (348.4804, 134.6578) -> (348.4328, 134.6868)
  line L640 (325.0424, 117.6225) -> (325.0569, 117.6768)
  line L641 (348.6166, 134.561) -> (348.5723, 134.5948)
  line L642 (348.3843, 134.7142) -> (348.3349, 134.7399)
  line L643 (348.5269, 134.6271) -> (348.4804, 134.6578)
  line L644 (349.1916, 133.6323) -> (349.1791, 133.6866)
  line L645 (348.076, 134.8419) -> (348.0223, 134.8569)
  line L646 (349.1791, 133.6866) -> (349.1648, 133.7405)
  line L647 (349.2223, 133.4118) -> (349.2175, 133.4673)
  line L648 (349.1486, 133.7938) -> (349.1306, 133.8465)
  line L649 (349.0138, 134.0991) -> (348.9853, 134.147)
  line L650 (325.0803, 117.7866) -> (325.0891, 117.842)
  line L651 (348.742, 134.4506) -> (348.7015, 134.4888)
  line L652 (348.6596, 134.5256) -> (348.6166, 134.561)
  line L653 (346.187, 134.0338) -> (346.1624, 133.9838)
  line L654 (347.9524, 131.7275) -> (348.0071, 131.7401)
  line L655 (346.5211, 134.4762) -> (346.481, 134.4375)
  line L656 (346.1186, 133.8813) -> (346.0994, 133.829)
  line L657 (346.0486, 132.9503) -> (346.0616, 132.8962)
  line L658 (346.2317, 132.4857) -> (346.2607, 132.4381)
  line L659 (347.1424, 134.8365) -> (347.0895, 134.8191)
  line L660 (347.3044, 134.8776) -> (347.2499, 134.8658)
  line L661 (346.0169, 133.4488) -> (346.0127, 133.3932)
  line L662 (346.5625, 134.5135) -> (346.5211, 134.4762)
  line L663 (346.2914, 132.3916) -> (346.3237, 132.3462)
  line L664 (346.0127, 133.3932) -> (346.0104, 133.3376)
  line L665 (346.3575, 132.3019) -> (346.3929, 132.2589)
  line L666 (346.1324, 132.685) -> (346.1546, 132.6339)
  line L667 (346.0664, 133.7226) -> (346.0527, 133.6686)
  line L668 (346.0616, 132.8962) -> (346.0766, 132.8425)
  line L669 (346.0281, 133.0599) -> (346.0374, 133.0049)
  line L670 (346.0409, 133.6141) -> (346.031, 133.5593)
  line L671 (346.0207, 133.1151) -> (346.0281, 133.0599)
  line L672 (346.4297, 132.217) -> (346.4679, 132.1765)
  line L673 (346.4679, 132.1765) -> (346.5076, 132.1374)
  line L674 (346.0994, 133.829) -> (346.082, 133.7761)
  line L675 (346.405, 134.356) -> (346.3691, 134.3134)
  line L676 (346.5076, 132.1374) -> (346.5485, 132.0996)
  line L677 (346.302, 134.2245) -> (346.2708, 134.1783)
  line L678 (346.2412, 134.1311) -> (346.2132, 134.0829)
  line L679 (346.3929, 132.2589) -> (346.4297, 132.217)
  line L680 (346.031, 133.5593) -> (346.023, 133.5042)
  line L681 (346.0117, 133.2261) -> (346.0152, 133.1705)
  line L682 (346.1624, 133.9838) -> (346.1396, 133.9329)
  line L683 (346.4423, 134.3974) -> (346.405, 134.356)
  line L684 (346.0101, 133.2818) -> (346.0117, 133.2261)
  line L685 (346.2132, 134.0829) -> (346.187, 134.0338)
  line L686 (346.2607, 132.4381) -> (346.2914, 132.3916)
  line L687 (347.0895, 134.8191) -> (347.0372, 134.7999)
  line L688 (346.0152, 133.1705) -> (346.0207, 133.1151)
  line L689 (346.7402, 134.6477) -> (346.694, 134.6165)
  line L690 (346.3348, 134.2695) -> (346.302, 134.2245)
  line L691 (346.0934, 132.7894) -> (346.112, 132.7369)
  line L692 (346.0104, 133.3376) -> (346.0101, 133.2818)
  line L693 (346.8847, 134.7315) -> (346.8356, 134.7053)
  line L694 (346.0374, 133.0049) -> (346.0486, 132.9503)
  line L695 (346.7874, 134.6773) -> (346.7402, 134.6477)
  line L696 (346.112, 132.7369) -> (346.1324, 132.685)
  line L697 (346.8356, 134.7053) -> (346.7874, 134.6773)
  line L698 (346.3237, 132.3462) -> (346.3575, 132.3019)
  line L699 (346.023, 133.5042) -> (346.0169, 133.4488)
  line L700 (346.649, 134.5837) -> (346.6051, 134.5494)
  line L701 (347.1959, 134.8521) -> (347.1424, 134.8365)
  line L702 (346.9347, 134.7561) -> (346.8847, 134.7315)
  line L703 (346.481, 134.4375) -> (346.4423, 134.3974)
  line L704 (346.1396, 133.9329) -> (346.1186, 133.8813)
  line L705 (346.2043, 132.5342) -> (346.2317, 132.4857)
  line L706 (346.694, 134.6165) -> (346.649, 134.5837)
  line L707 (346.9856, 134.7789) -> (346.9347, 134.7561)
  line L708 (346.1546, 132.6339) -> (346.1786, 132.5836)
  line L709 (346.2708, 134.1783) -> (346.2412, 134.1311)
  line L710 (346.0527, 133.6686) -> (346.0409, 133.6141)
  line L711 (346.1786, 132.5836) -> (346.2043, 132.5342)
  line L712 (346.3691, 134.3134) -> (346.3348, 134.2695)
  line L713 (347.2499, 134.8658) -> (347.1959, 134.8521)
  line L714 (346.6051, 134.5494) -> (346.5625, 134.5135)
  line L715 (346.0766, 132.8425) -> (346.0934, 132.7894)
  line L716 (346.5485, 132.0996) -> (346.5908, 132.0632)
  line L717 (349.1475, 132.8035) -> (349.1639, 132.8572)
  line L718 (348.6518, 132.0685) -> (348.6941, 132.1054)
  line L719 (349.1639, 132.8572) -> (349.1784, 132.9114)
  line L720 (346.5908, 132.0632) -> (346.6342, 132.0284)
  line L721 (346.9685, 131.8293) -> (347.0199, 131.8077)
  line L722 (347.2319, 131.7394) -> (347.2862, 131.7269)
  line L723 (347.2862, 131.7269) -> (347.3409, 131.7164)
  line L724 (349.1911, 132.9661) -> (349.2018, 133.0212)
  line L725 (347.1247, 131.7699) -> (347.178, 131.7537)
  line L726 (348.6081, 132.0332) -> (348.6518, 132.0685)
  line L727 (347.6181, 131.6923) -> (347.6742, 131.6933)
  line L728 (348.8131, 132.2244) -> (348.85, 132.2667)
  line L729 (348.6941, 132.1054) -> (348.7352, 132.1436)
  line L730 (347.0199, 131.8077) -> (347.072, 131.7879)
  line L731 (348.5633, 131.9994) -> (348.6081, 132.0332)
  line L732 (348.85, 132.2667) -> (348.8853, 132.3104)
  line L733 (347.5067, 131.6962) -> (347.5624, 131.6933)
  line L734 (347.7862, 131.7011) -> (347.8419, 131.708)
  line L735 (348.7749, 132.1833) -> (348.8131, 132.2244)
  line L736 (349.0634, 132.5955) -> (349.0872, 132.6463)
  line L737 (347.3409, 131.7164) -> (347.3959, 131.7077)
  line L738 (348.0071, 131.7401) -> (348.0613, 131.7546)
  line L739 (349.1784, 132.9114) -> (349.1911, 132.9661)
  line L740 (346.8682, 131.8778) -> (346.918, 131.8527)
  line L741 (349.0107, 132.4964) -> (349.038, 132.5455)
  line L742 (348.323, 131.8551) -> (348.373, 131.8805)
  line L743 (348.7352, 132.1436) -> (348.7749, 132.1833)
  line L744 (348.115, 131.771) -> (348.1681, 131.7893)
  line L745 (346.8194, 131.9047) -> (346.8682, 131.8778)
  line L746 (348.4221, 131.9078) -> (348.4703, 131.9367)
  line L747 (348.5173, 131.9672) -> (348.5633, 131.9994)
  line L748 (348.2722, 131.8313) -> (348.323, 131.8551)
  line L749 (346.6789, 131.9951) -> (346.7247, 131.9633)
  line L750 (349.1292, 132.7504) -> (349.1475, 132.8035)
  line L751 (349.2018, 133.0212) -> (349.2105, 133.0766)
  line L752 (348.8853, 132.3104) -> (348.9191, 132.3552)
  line L753 (347.3959, 131.7077) -> (347.4512, 131.701)
  line L754 (347.5624, 131.6933) -> (347.6181, 131.6923)
  line L755 (349.2105, 133.0766) -> (349.2174, 133.1323)
  line L756 (349.038, 132.5455) -> (349.0634, 132.5955)
  line L757 (347.178, 131.7537) -> (347.2319, 131.7394)
  line L758 (347.072, 131.7879) -> (347.1247, 131.7699)
  line L759 (348.373, 131.8805) -> (348.4221, 131.9078)
  line L760 (347.8973, 131.7167) -> (347.9524, 131.7275)
  line L761 (348.2205, 131.8094) -> (348.2722, 131.8313)
  line L762 (348.4703, 131.9367) -> (348.5173, 131.9672)
  line L763 (347.6742, 131.6933) -> (347.7303, 131.6962)
  line L764 (347.7303, 131.6962) -> (347.7862, 131.7011)
  line L765 (348.9513, 132.4012) -> (348.9818, 132.4482)
  line L766 (346.7715, 131.9332) -> (346.8194, 131.9047)
  line L767 (348.9818, 132.4482) -> (349.0107, 132.4964)
  line L768 (346.6342, 132.0284) -> (346.6789, 131.9951)
  line L769 (346.918, 131.8527) -> (346.9685, 131.8293)
  line L770 (346.7247, 131.9633) -> (346.7715, 131.9332)
  line L771 (347.4512, 131.701) -> (347.5067, 131.6962)
  line L772 (348.0613, 131.7546) -> (348.115, 131.771)
  line L773 (348.1681, 131.7893) -> (348.2205, 131.8094)
  line L774 (348.9191, 132.3552) -> (348.9513, 132.4012)
  line L775 (349.0872, 132.6463) -> (349.1091, 132.698)
  line L776 (349.1091, 132.698) -> (349.1292, 132.7504)
  line L777 (353.4161, 86.5973) -> (353.3638, 86.5781)
  line L778 (354.4557, 86.6034) -> (354.4026, 86.6201)
  line L779 (353.2613, 86.5343) -> (353.2113, 86.5098)
  line L780 (354.2402, 86.6593) -> (354.1852, 86.6686)
  line L781 (354.7594, 86.465) -> (354.7109, 86.4924)
  line L782 (354.0746, 86.6815) -> (354.019, 86.685)
  line L783 (354.8535, 86.4053) -> (354.807, 86.436)
  line L784 (353.8519, 86.684) -> (353.7963, 86.6799)
  line L785 (355.1077, 86.1891) -> (355.0686, 86.2288)
  line L786 (355.5374, 85.3008) -> (355.5287, 85.3558)
  line L787 (355.3119, 85.9252) -> (355.2818, 85.972)
  line L788 (354.019, 86.685) -> (353.9633, 86.6866)
  line L789 (353.469, 86.6147) -> (353.4161, 86.5973)
  line L790 (354.807, 86.436) -> (354.7594, 86.465)
  line L791 (354.9862, 86.3038) -> (354.9432, 86.3392)
  line L792 (355.3673, 85.8285) -> (355.3404, 85.8773)
  line L793 (355.4752, 85.572) -> (355.4572, 85.6247)
  line L794 (349.2174, 133.1323) -> (349.2223, 133.1882)
  line L795 (353.3122, 86.5571) -> (353.2613, 86.5343)
  line L796 (355.5441, 85.2455) -> (355.5374, 85.3008)
  line L797 (355.4374, 85.6768) -> (355.4158, 85.7282)
  line L798 (355.1819, 86.1059) -> (355.1455, 86.1482)
  line L799 (355.0686, 86.2288) -> (355.0281, 86.267)
  line L800 (355.4158, 85.7282) -> (355.3924, 85.7787)
  line L801 (347.8419, 131.708) -> (347.8973, 131.7167)
  line L802 (353.7409, 86.6738) -> (353.6858, 86.6657)
  line L803 (353.5225, 86.6303) -> (353.469, 86.6147)
  line L804 (355.3404, 85.8773) -> (355.3119, 85.9252)
  line L805 (353.7963, 86.6799) -> (353.7409, 86.6738)
  line L806 (355.0281, 86.267) -> (354.9862, 86.3038)
  line L807 (355.5057, 85.4648) -> (355.4914, 85.5187)
  line L808 (354.8989, 86.373) -> (354.8535, 86.4053)
  line L809 (354.5601, 86.5643) -> (354.5082, 86.5847)
  line L810 (355.3924, 85.7787) -> (355.3673, 85.8285)
  line L811 (353.9633, 86.6866) -> (353.9075, 86.6863)
  line L812 (353.9075, 86.6863) -> (353.8519, 86.684)
  line L813 (355.2167, 86.0625) -> (355.1819, 86.1059)
  line L814 (354.13, 86.676) -> (354.0746, 86.6815)
  line L815 (353.6858, 86.6657) -> (353.631, 86.6558)
  line L816 (353.2113, 86.5098) -> (353.1622, 86.4835)
  line L817 (355.2818, 85.972) -> (355.25, 86.0178)
  line L818 (355.5489, 85.19) -> (355.5441, 85.2455)
  line L819 (355.5182, 85.4105) -> (355.5057, 85.4648)
  line L820 (354.2948, 86.6481) -> (354.2402, 86.6593)
  line L821 (349.2252, 133.2443) -> (349.2262, 133.3004)
  line L822 (355.4572, 85.6247) -> (355.4374, 85.6768)
  line L823 (355.5528, 85.0786) -> (355.5518, 85.1343)
  line L824 (354.1852, 86.6686) -> (354.13, 86.676)
  line L825 (349.2223, 133.1882) -> (349.2252, 133.2443)
  line L826 (352.9174, 83.8415) -> (352.9608, 83.8066)
  line L827 (352.8477, 86.2544) -> (352.8076, 86.2157)
  line L828 (353.0981, 83.7114) -> (353.146, 83.6829)
  line L829 (353.146, 83.6829) -> (353.1948, 83.656)
  line L830 (352.7195, 84.0371) -> (352.7563, 83.9952)
  line L831 (353.5765, 86.644) -> (353.5225, 86.6303)
  line L832 (352.3882, 84.6744) -> (352.4032, 84.6207)
  line L833 (352.4812, 84.4121) -> (352.5052, 84.3618)
  line L834 (354.6615, 86.5181) -> (354.6112, 86.5421)
  line L835 (355.4914, 85.5187) -> (355.4752, 85.572)
  line L836 (355.5518, 85.1343) -> (355.5489, 85.19)
  line L837 (355.1455, 86.1482) -> (355.1077, 86.1891)
  line L838 (353.3638, 86.5781) -> (353.3122, 86.5571)
  line L839 (355.5287, 85.3558) -> (355.5182, 85.4105)
  line L840 (354.4026, 86.6201) -> (354.3489, 86.6351)
  line L841 (355.25, 86.0178) -> (355.2167, 86.0625)
  line L842 (354.3489, 86.6351) -> (354.2948, 86.6481)
  line L843 (353.0513, 83.7415) -> (353.0981, 83.7114)
  line L844 (352.3418, 84.9487) -> (352.3473, 84.8933)
  line L845 (353.631, 86.6558) -> (353.5765, 86.644)
  line L846 (353.1948, 83.656) -> (353.2446, 83.6309)
  line L847 (352.8076, 86.2157) -> (352.7689, 86.1756)
  line L848 (353.2446, 83.6309) -> (353.2951, 83.6075)
  line L849 (354.9432, 86.3392) -> (354.8989, 86.373)
  line L850 (354.7109, 86.4924) -> (354.6615, 86.5181)
  line L851 (354.5082, 86.5847) -> (354.4557, 86.6034)
  line L852 (354.6112, 86.5421) -> (354.5601, 86.5643)
  line L853 (352.9608, 83.8066) -> (353.0055, 83.7733)
  line L854 (353.0055, 83.7733) -> (353.0513, 83.7415)
  line L855 (352.9756, 86.3619) -> (352.9317, 86.3276)
  line L856 (352.5974, 85.9565) -> (352.5678, 85.9093)
  line L857 (352.3675, 85.3923) -> (352.3576, 85.3375)
  line L858 (352.337, 85.1158) -> (352.3367, 85.06)
  line L859 (352.5052, 84.3618) -> (352.5309, 84.3124)
  line L860 (353.0668, 86.4259) -> (353.0206, 86.3947)
  line L861 (352.426, 85.6072) -> (352.4086, 85.5543)
  line L862 (352.9317, 86.3276) -> (352.8891, 86.2917)
  line L863 (352.3473, 84.8933) -> (352.3547, 84.8381)
  line L864 (352.3435, 85.227) -> (352.3393, 85.1714)
  line L865 (352.8751, 83.8778) -> (352.9174, 83.8415)
  line L866 (354.7969, 83.7149) -> (354.8439, 83.7454)
  line L867 (355.1015, 83.9615) -> (355.1397, 84.0026)
  line L868 (353.114, 86.4555) -> (353.0668, 86.4259)
  line L869 (352.3383, 85.0043) -> (352.3418, 84.9487)
  line L870 (352.5136, 85.812) -> (352.489, 85.762)
  line L871 (352.7689, 86.1756) -> (352.7316, 86.1342)
  line L872 (352.4452, 85.6595) -> (352.426, 85.6072)
  line L873 (352.364, 84.7831) -> (352.3752, 84.7285)
  line L874 (352.5583, 84.2639) -> (352.5873, 84.2163)
  line L875 (352.3752, 84.7285) -> (352.3882, 84.6744)
  line L876 (352.42, 84.5676) -> (352.4386, 84.5151)
  line L877 (352.6957, 86.0916) -> (352.6614, 86.0477)
  line L878 (352.6841, 84.0801) -> (352.7195, 84.0371)
  line L879 (352.5678, 85.9093) -> (352.5398, 85.8611)
  line L880 (352.459, 84.4632) -> (352.4812, 84.4121)
  line L881 (352.4086, 85.5543) -> (352.393, 85.5008)
  line L882 (352.8342, 83.9156) -> (352.8751, 83.8778)
  line L883 (352.5398, 85.8611) -> (352.5136, 85.812)
  line L884 (352.3547, 84.8381) -> (352.364, 84.7831)
  line L885 (352.4032, 84.6207) -> (352.42, 84.5676)
  line L886 (352.6503, 84.1244) -> (352.6841, 84.0801)
  line L887 (352.6614, 86.0477) -> (352.6286, 86.0027)
  line L888 (352.489, 85.762) -> (352.4662, 85.7111)
  line L889 (352.393, 85.5008) -> (352.3793, 85.4468)
  line L890 (352.5873, 84.2163) -> (352.618, 84.1698)
  line L891 (352.7316, 86.1342) -> (352.6957, 86.0916)
  line L892 (352.8891, 86.2917) -> (352.8477, 86.2544)